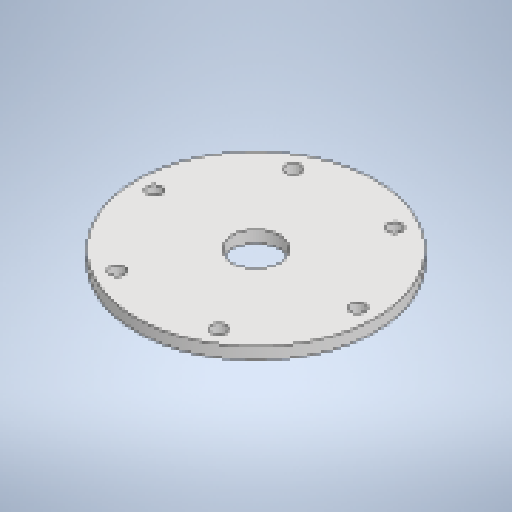
# Autodesk Inventor part: NVPH-412 cup head flange
Saved by Autodesk Inventor 2025.1 (Build 291241020, 241B)
## iProperties
Created: 2024-12-03
Part Number: NVPH-412 cup head flange
Material: Generic
Document SubType Name: Sheet Metal
Designer: user
Density: 1 g/cm^3
Flat Pattern Width: 20 cm
Flat Pattern Length: 20 cm
Flat Pattern Area: 400 cm^2
Sheet Metal Rule: Default_mm
Sheet Metal Width: 200.000 mm
Sheet Metal Length: 200.000 mm
Sheet Metal Area: 40000.000 mm^2
Appearance: Default
Author: user
Autodesk Inventor part; units mm, degrees
ref_plane "YZ Plane" through (0, 0, 0) normal (1, 0, 0) x (0, 1, 0)
ref_plane "XZ Plane" through (0, 0, 0) normal (0, 1, 0) x (-1, 0, 0)
ref_plane "XY Plane" through (0, 0, 0) normal (0, 0, 1) x (1, 0, 0)
sketch "Sketch1" plane through (0, 0, 0) normal (0, 0, 1) x (1, 0, 0)
  circle A0 centre (0, 0) radius 20
  circle A1 centre (0, 0) radius 100
  dimension "d0" = 40
  dimension "d1" = 200
  constraints: 2 centre point, 2 coincident
  measures "d0" diameter of A0
  measures "d1" diameter of A1
extrude "Extrusion1" add sketch "Sketch1" against normal blind 10
sketch "Sketch3" plane through (0, 0, 0) normal (0, 0, 1) x (1, 0, 0)
  circle A0 centre (80, 0) radius 6
  circle A1 centre (0, 0) radius 80 construction
  dimension "d4" = 160
  dimension "d5" = 12
  constraints: 2 horizontal alignment, 1 centre point, 1 coincident, 2 other
  measures "d5" diameter of A0
extrude "Cut1" cut sketch "Sketch3" against normal blind 10
pattern_circular "Circular Pattern1" count 6 over 360 about axis through (0, 0, 0) along (0, 0, -1) of "Cut1"
equation "\"d7\" = Thickness"
equation "\"BendReliefDepth\" = 0.5 * Thickness"
equation "\"Thickness\" = 10"
body "Solid1"
